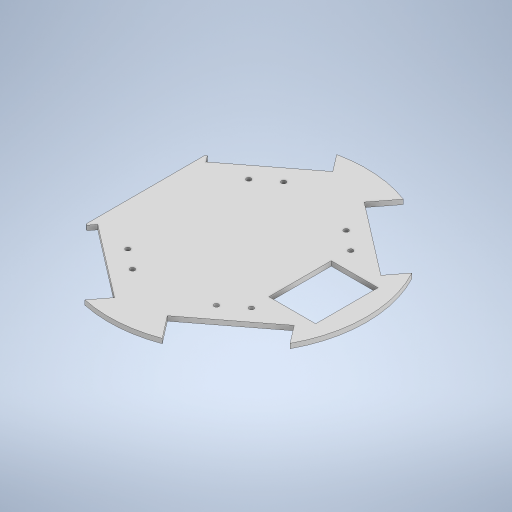
# Autodesk Inventor part: newbasecentral
Saved by Autodesk Inventor 2023.1 (Build 271208000, 208)
## iProperties
Created: 2022-09-07
Part Number: newbasecentral
Material: Genérico
Document SubType Name: Modeling
Designer: Lab. de Manufactura
Density: 1 g/cm^3
Appearance: Valor por defecto
Author: Lab. de Manufactura
Autodesk Inventor part; units mm, degrees
ref_plane "YZ Plane" through (0, 0, 0) normal (1, 0, 0) x (0, 1, 0)
ref_plane "XZ Plane" through (0, 0, 0) normal (0, 1, 0) x (-1, 0, 0)
ref_plane "XY Plane" through (0, 0, 0) normal (0, 0, 1) x (1, 0, 0)
sketch "Boceto1" plane through (0, 0, 0) normal (0, 1, 0) x (-1, 0, 0)
  line L0 (0, 0) -> (0, -52.2241) construction
  line L1 (0, 0) -> (0, 54.663) construction
  line L2 (0, 0) -> (-57.9564, 0) construction
  line L3 (0, 0) -> (56.3387, 0) construction
  line L4 (-70, -20) -> (-40, -20)
  line L5 (-40, -20) -> (-40, 20)
  line L6 (-40, 20) -> (-70, 20)
  line L7 (-70, 20) -> (-70, -20)
  line L8 (-70, -20) -> (-40, 20) construction
  line L9 (-40, -20) -> (-70, 20) construction
  line L10 (-18, 63.0769) -> (-64.0145, 27.7688)
  line L11 (9, 69.9829) -> (55.0145, 34.6747)
  line L12 (9, 69.9829) -> (17.2117, 80.6846)
  line L13 (-18, 63.0769) -> (-28.8943, 77.2746)
  line L14 (-64.0145, 27.7688) -> (-72.6721, 39.0515)
  line L15 (-18, -63.0769) -> (-64.0145, -27.7688)
  line L16 (9, -69.9829) -> (55.0145, -34.6747)
  line L17 (9, -69.9829) -> (17.2117, -80.6846)
  line L18 (-18, -63.0769) -> (-28.8943, -77.2746)
  line L19 (-64.0145, -27.7688) -> (-72.6721, -39.0515)
  arc A0 (-72.6721, 39.0515) -> (-72.6721, -39.0515) centre (0, 0) ccw
  arc A1 (17.2117, 80.6846) -> (-28.8943, 77.2746) centre (0, 0) ccw
  arc A2 (-28.8943, -77.2746) -> (17.2117, -80.6846) centre (0, 0) ccw
  line L20 (59, 37.9189) -> (59, -37.9189)
  line L21 (58.0583, 38.6415) -> (59, 37.9189)
  line L22 (55.0145, 34.6747) -> (58.0583, 38.6415)
  line L23 (58.0583, -38.6415) -> (59, -37.9189)
  line L24 (55.0145, -34.6747) -> (58.0583, -38.6415)
  circle A3 centre (-27.964, 41.5661) radius 1.5
  circle A4 centre (-40.6577, 31.8259) radius 1.5
  line L25 (-41.0072, 45.4229) -> (-34.3109, 36.696) construction
  line L26 (-27.964, 41.5661) -> (-40.6577, 31.8259) construction
  line L27 (32.0072, 52.3288) -> (22.9685, 40.5493) construction
  circle A5 centre (18.964, 48.472) radius 1.5
  circle A6 centre (31.6577, 38.7318) radius 1.5
  circle A7 centre (-27.964, -41.5661) radius 1.5
  circle A8 centre (-40.6577, -31.8259) radius 1.5
  circle A9 centre (18.964, -48.472) radius 1.5
  circle A10 centre (31.6577, -38.7318) radius 1.5
  point P0 (-55, 0)
  point P1 (-70, 0)
  dimension "d1" = 30
  dimension "d2" = 40
  dimension "d3" = 70
  dimension "d9" = 52.5
  dimension "d10" = 52.5
  dimension "d11" = 61
  dimension "d12" = 61
  dimension "d13" = 58
  dimension "d17" = 90
  dimension "d18" = 9
  dimension "d19" = 18
  dimension "d20" = 58
  dimension "d21" = 90
  dimension "d22" = 90
  dimension "d23" = 82.5
  dimension "d24" = 82.5
  dimension "d26" = 59
  dimension "d27" = 5
  dimension "d28" = 5
  dimension "d29" = 3
  dimension "d30" = 3
  dimension "d31" = 16
  dimension "d32" = 11
  dimension "d33" = 11
  dimension "d37" = 90
  dimension "d38" = 3
  dimension "d39" = 3
  dimension "d40" = 16
  dimension "d41" = 11
  dimension "d42" = 11
  dimension "d43" = 8
  constraints: 56 end point, 11 centre point, 11 symmetric about line, 7 parallel, 6 midpoint, 6 point on circle, 3 horizontal, 3 vertical, 2 perpendicular, 1 coincident, 1 point on line, 4 other
  measures "d1" distance of L5.end L6.end
  measures "d2" distance of L4.end L5.end
  measures "d3" distance of L0.start point (-70, 0)
  measures "d9" angle of L1 L11
  measures "d10" angle of L1 L10
  measures "d11" distance from line of point (0, 0) L11
  measures "d12" distance from line of point (0, 0) L10
  measures "d13" distance of L11.start L11.end
  measures "d17" angle of L11 L12
  measures "d18" distance from line of L1 L11.start
  measures "d19" distance from line of L1 L10.start
  measures "d20" distance of L10.start L10.end
  measures "d21" angle of L10 L13
  measures "d22" angle of L10 L14
  measures "d23" radius of A0
  measures "d24" radius of A1
  measures "d26" distance between parallel lines of L0 L20
  measures "d27" distance between parallel lines of L11 L21
  measures "d28" distance between parallel lines of L23 L16
  measures "d29" diameter of A3
  measures "d30" diameter of A4
  measures "d31" distance of L26.end L26.start
  measures "d32" distance from line of L10 L26.start
  measures "d33" distance from line of L10 L26.end
  measures "d37" angle of L11 L27
  measures "d38" diameter of A5
  measures "d39" diameter of A6
  measures "d40" distance of A5.centre A6.centre
  measures "d41" distance from line of L11 A5.centre
  measures "d42" distance from line of L11 A6.centre
  measures "d43" distance from line of L27 A5.centre
extrude "Extrusión1" add sketch "Boceto1" along normal blind 3
